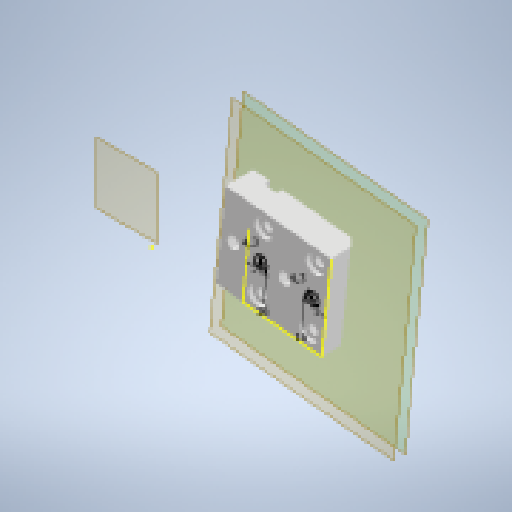
# Autodesk Inventor part: полное крепление каретки
Saved by Autodesk Inventor 2024.2 (Build 282272000, 272)
## iProperties
Created: 2026-01-10
Part Number: полное крепление каретки
Material: Типовые
Document SubType Name: Modeling
Designer: Service
Density: 1 g/cm^3
Appearance: По умолчанию
Author: Service
Autodesk Inventor part; units mm, degrees
ref_plane "YZ Plane" through (0, 0, 0) normal (1, 0, 0) x (0, 1, 0)
ref_plane "XZ Plane" through (0, 0, 0) normal (0, 1, 0) x (-1, 0, 0)
ref_plane "XY Plane" through (0, 0, 0) normal (0, 0, 1) x (1, 0, 0)
ref_plane "РабПлоскость1" through (48.6356, 13.505, -4) normal (0, 0, -1) x (0.7272082, -0.6864169, 0)
ref_plane "РабПлоскость2" through (48.6356, 13.505, 0) normal (0, 0, 1) x (-0.7272082, 0.6864169, 0)
sketch "Эскиз2" plane through (48.6356, 13.505, 0) normal (0, 0, 1) x (-0.7272082, 0.6864169, 0)
  line L0 (-17.8008, -6.6339) -> (10.6717, -6.6339)
  line L1 (10.6717, -6.6339) -> (10.6717, 25.3661)
  line L2 (10.6717, 25.3661) -> (-17.8008, 25.3661)
  line L3 (-17.8008, 25.3661) -> (-17.8008, -6.6339)
  circle A0 centre (-31.4768, 2.1354) radius 0.9
  circle A1 centre (23.5157, 1.4536) radius 0.9
  circle A2 centre (-19.4778, 1.9866) radius 0.9
  circle A3 centre (-19.5769, -6.0128) radius 0.9
  circle A4 centre (23.4165, -6.5458) radius 0.9
  circle A5 centre (11.5166, 1.6023) radius 0.9
  circle A6 centre (11.4174, -6.3971) radius 0.9
  circle A7 centre (-31.576, -5.864) radius 0.9
  circle A8 centre (-12.8008, -1.6339) radius 1.6
  circle A9 centre (5.6717, -1.6339) radius 1.6
  circle A10 centre (-12.8008, 20.3661) radius 1.6
  circle A11 centre (5.6717, 20.3661) radius 1.6
  arc A12 (11.4355, 36.4061) -> (11.4355, 44.3661) centre (11.4355, 40.3861) ccw
  line L4 (11.4355, 44.3661) -> (-18.5645, 44.3661)
  arc A13 (-18.5645, 44.3661) -> (-18.5645, 36.4061) centre (-18.5645, 40.3861) ccw
  line L5 (-18.5645, 36.4061) -> (11.4355, 36.4061)
  line L6 (-33.5645, -20.6339) -> (-33.5645, 49.3661)
  line L7 (-33.5645, 49.3661) -> (26.4355, 49.3661)
  line L8 (26.4355, 49.3661) -> (26.4355, -20.6339)
  line L9 (26.4355, -20.6339) -> (-33.5645, -20.6339)
  circle A14 centre (-12.8008, 9.3661) radius 2.15
  circle A15 centre (5.6717, 9.3661) radius 2.15
  point P0 (26.0981, 43.2052)
  point P1 (-17.8008, 9.3661)
  point P2 (10.5491, -6.6339)
  point P3 (10.6717, -5.8931)
  point P4 (10.6717, 1.2922)
  point P5 (10.6717, 1.9125)
  dimension "d0" = 5
  dimension "d1" = 5
  dimension "d2" = 5
  dimension "d3" = 5
  dimension "d4" = 4.3
  dimension "d5" = 4.3
  dimension "d6" = 16
  dimension "d7" = 5
  dimension "d8" = 16
  dimension "d9" = 5
  constraints: 20 end point, 16 centre point, 5 horizontal, 4 point on circle, 2 parallel, 2 vertical, 1 midpoint, 1 perpendicular, 36 other
  measures "d0" distance from line of L3 A10.centre
  measures "d1" distance from line of L0 A8.centre
  measures "d2" distance from line of L1 A9.centre
  measures "d3" distance from line of L2 A11.centre
  measures "d4" diameter of A15
  measures "d5" diameter of A14
  measures "d6" distance from line of L2 A14.centre
  measures "d7" distance from line of L1 A15.centre
  measures "d8" distance from line of L0 A15.centre
  measures "d9" distance of point (-17.801, 9.366) A14.centre
extrude "Выдавливание1" add sketch "Эскиз2" along normal blind 10 contours L3 L2 L1 A5 A6 L0 | A14 | A15
sketch "Эскиз3" plane through (48.6356, 13.505, 10) normal (0, 0, 1) x (-0.7272082, 0.6864169, 0)
  circle A0 centre (-12.8008, 9.3661) radius 2.15
  circle A1 centre (5.6717, 9.3661) radius 2.15
  line L0 (10.6717, 1.9125) -> (10.6717, 25.3661) projected
  line L1 (10.6717, 25.3661) -> (-17.8008, 25.3661) projected
  line L2 (-17.8008, 25.3661) -> (-17.8008, -6.6339) projected
  point P0 (26.0981, 43.2052)
  dimension "d12" = 5
  dimension "d13" = 16
  dimension "d14" = 5
  dimension "d15" = 16
  dimension "d16" = 4.3
  dimension "d17" = 4.3
  constraints: 2 centre point
  measures "d12" distance from line of L0 A1.centre
  measures "d13" distance from line of L1 A1.centre
  measures "d14" distance from line of L2 A0.centre
  measures "d15" distance from line of L1 A0.centre
  measures "d16" diameter of A0
  measures "d17" diameter of A1
ref_plane "РабПлоскость3" through (-12.8008, 9.3661, 6) normal (0, 0, 1) x (1, 0, 0)
sketch "Эскиз4" plane through (-12.8008, 9.3661, 6) normal (0, 0, 1) x (1, 0, 0)
  line L0 (-12.8791, 27.3861) -> (32.0773, 27.3861)
  line L1 (32.0773, 27.3861) -> (32.0773, -22.3728)
  line L2 (32.0773, -22.3728) -> (-12.8791, -22.3728)
  line L3 (-12.8791, -22.3728) -> (-12.8791, 27.3861)
  point P0 (12.8008, -9.3661)
  constraints: 8 end point, 2 parallel, 1 horizontal, 1 perpendicular
extrude "Выдавливание3" cut sketch "Эскиз4" against normal blind 10
sketch "Эскиз5" plane through (48.6356, 13.505, 10) normal (0, 0, 1) x (-0.7272082, 0.6864169, 0)
  line L0 (-17.8008, -6.6339) -> (10.5491, -6.6339) projected
  arc A0 (10.6717, -5.8931) -> (10.5491, -6.6339) centre (11.4174, -6.3971) ccw projected
  line L1 (10.6717, -5.8931) -> (10.6717, 1.2922) projected
  arc A1 (10.6717, 1.9125) -> (10.6717, 1.2922) centre (11.5166, 1.6023) ccw projected
  line L2 (10.6717, 1.9125) -> (10.6717, 25.3661) projected
  line L3 (10.6717, 25.3661) -> (-17.8008, 25.3661) projected
  line L4 (-17.8008, 25.3661) -> (-17.8008, -6.6339) projected
  circle A2 centre (5.6717, 20.3661) radius 1.6 projected
  circle A3 centre (5.6717, -1.6339) radius 1.6 projected
  circle A4 centre (-12.8008, -1.6339) radius 1.6 projected
  circle A5 centre (-12.8008, 20.3661) radius 1.6 projected
  circle A6 centre (-12.8008, -1.6339) radius 3.25
  circle A7 centre (5.6717, -1.6339) radius 3.25
  circle A8 centre (5.6717, 20.3661) radius 3.25
  circle A9 centre (-12.8008, 20.3661) radius 3.25
  point P0 (26.0981, 43.2052)
  dimension "d22" = 6.5
  constraints: 4 centre point, 4 coincident, 3 equal radius
  measures "d22" diameter of A9
extrude "Выдавливание4" cut sketch "Эскиз5" against normal blind 1.5 contours A2 | A3 | A6 | A7 | A8 | A9
sketch "Эскиз6" plane through (48.6356, 13.505, 10) normal (0, 0, 1) x (-0.7272082, 0.6864169, 0)
  circle A0 centre (-2.8008, 9.3661) radius 2.15
  circle A1 centre (15.6717, 9.3661) radius 2.15
  circle A2 centre (-12.8008, 9.3661) radius 2.15 projected
  circle A3 centre (5.6717, 9.3661) radius 2.15 projected
  line L0 (-12.8008, 9.3661) -> (5.6717, 9.3661) construction
  point P0 (26.0981, 43.2052)
  dimension "d25" = 10
  dimension "d27" = 10
  constraints: 2 centre point, 2 end point, 2 equal radius, 2 point on line, 1 horizontal
  measures "d25" distance of L0.end A1.centre
  measures "d27" distance of L0.start A0.centre
sketch "Эскиз7" plane through (48.6356, 13.505, 10) normal (0, 0, 1) x (-0.7272082, 0.6864169, 0)
  line L0 (-17.8008, -6.6339) -> (10.5491, -6.6339) projected
  line L1 (10.5491, -6.6339) -> (20, -6.6339)
  line L2 (20, -6.6339) -> (20, 25.3661)
  line L3 (20, 25.3661) -> (10.5491, 25.3661)
  line L4 (10.5491, 25.3661) -> (10.5491, -6.6339)
  point P0 (26.0981, 43.2052)
  constraints: 8 end point, 2 parallel, 1 horizontal, 1 perpendicular
extrude "Выдавливание5" add sketch "Эскиз7" against normal up to surface (10 mm away)
extrude "Выдавливание6" cut sketch "Эскиз6" against normal blind 3 contours A0 | A1
chamfer "Фаска1" distance 3 angle 45 1 edges at (55.1514, -5.5248, 0)
sketch "Эскиз8" plane through (38.645, 32.0576, 10) normal (0.6864169, 0.7272082, 0) x (0.7272082, -0.6864169, 0)
  line L0 (34.8008, 10) -> (9.4509, 10) projected
  line L1 (10.3048, 10) -> (6, 10)
  line L2 (6, 10) -> (6, 8)
  line L3 (6, 8) -> (10.3048, 8)
  line L4 (10.3048, 8) -> (10.3048, 10)
  point P0 (-6.0981, 10)
  point P1 (9.4509, 10)
  point P2 (13.424, 10)
  constraints: 8 end point, 2 parallel, 1 horizontal, 1 perpendicular, 1 point on line
extrude "Выдавливание7" cut sketch "Эскиз8" against normal through all
